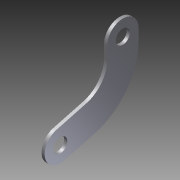
# Autodesk Inventor part: Claw
Saved by Autodesk Inventor 2012 (Build 160160000, 160)
## iProperties
Created: 2011-09-11
Part Number: Claw
Material: Default
Document SubType Name: Modeling
Designer: Ian Walters
Density: 1 g/cm^3
Author: Ian Walters
Autodesk Inventor part; units mm, degrees
ref_plane "YZ Plane" through (0, 0, 0) normal (1, 0, 0) x (0, 1, 0)
ref_plane "XZ Plane" through (0, 0, 0) normal (0, 1, 0) x (-1, 0, 0)
ref_plane "XY Plane" through (0, 0, 0) normal (0, 0, 1) x (1, 0, 0)
sketch "Sketch2" plane through (0, 0, 0) normal (1, 0, 0) x (0, 0, -1)
  circle A0 centre (0, 0) radius 14.2875
  arc A1 (31.75, 0) -> (-31.75, 0) centre (0, 0) ccw
  line L0 (-31.75, 0) -> (-31.75, -25.4)
  line L1 (31.75, 0) -> (31.75, -25.4)
  arc A2 (-73.5669, -79.8968) -> (-31.75, -25.4) centre (-88.1693, -25.4) ccw
  arc A3 (-57.1319, -141.2331) -> (31.75, -25.4) centre (-88.1693, -25.4) ccw
  line L2 (-88.1693, -25.4) -> (-57.1319, -141.2331) construction
  line L3 (-73.5669, -79.8968) -> (-134.9032, -96.3319)
  line L4 (-57.1319, -141.2331) -> (-118.4682, -157.6681)
  arc A4 (-134.9032, -96.3319) -> (-118.4682, -157.6681) centre (-126.6857, -127) ccw
  circle A5 centre (-126.6857, -127) radius 14.2875
  line L5 (-88.1693, -25.4) -> (31.75, -25.4) construction
  dimension "d0" = 28.575
  dimension "d1" = 31.75
  dimension "d2" = 28.575
  dimension "d3" = 25.4
  dimension "d4" = 63.5
  dimension "d5" = 127
  dimension "d6" = 75
  constraints: 12 end point, 8 point on circle, 6 centre point, 6 tangent, 4 coincident, 4 parallel, 3 horizontal alignment, 2 perpendicular, 1 point on line, 1 vertical
  measures "d0" diameter of A0
  measures "d1" radius of A1
  measures "d2" diameter of A5
  measures "d3" distance of L1.start L1.end
  measures "d4" distance of L2.end L4.end
  measures "d5" vertical distance of point (0, 0) A4.centre
  measures "d6" angle of L5 L2
extrude "Extrusion1" add sketch "Sketch2" along normal blind 6.35
body "Solid1"
